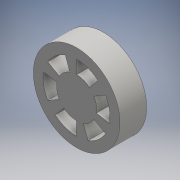
# Autodesk Inventor part: Large Flywheel
Saved by Autodesk Inventor 2016 (Build 200138000, 138)
## iProperties
Created: 2015-12-24
Part Number: Large Flywheel
Material: Generic
Document SubType Name: Modeling
Designer: jonathan
Density: 1 g/cm^3
Appearance: Default
Author: jonathan
Autodesk Inventor part; units mm, degrees
ref_plane "YZ Plane" through (0, 0, 0) normal (1, 0, 0) x (0, 1, 0)
ref_plane "XZ Plane" through (0, 0, 0) normal (0, 1, 0) x (-1, 0, 0)
ref_plane "XY Plane" through (0, 0, 0) normal (0, 0, 1) x (1, 0, 0)
sketch "Sketch1" plane through (0, 0, 0) normal (0, 1, 0) x (-1, 0, 0)
  circle A0 centre (0, 0) radius 65
  dimension "d0" = 130
  constraints: 1 centre point, 1 coincident
  measures "d0" diameter of A0
extrude "Extrusion1" add sketch "Sketch1" along normal blind 40
sketch "Sketch2" plane through (0, 0, 0) normal (0, -1, 0) x (1, 0, 0)
  line L0 (0, 0) -> (0, 50)
  arc A0 (32.1394, 38.3022) -> (0, 50) centre (0, 0) ccw
  arc A1 (19.2836, 22.9813) -> (0, 30) centre (0, 0) ccw
  line L1 (0, 0) -> (19.2836, 22.9813)
  line L2 (32.1394, 38.3022) -> (19.2836, 22.9813)
  dimension "d4" = 40
  dimension "d5" = 30
  dimension "d6" = 50
  constraints: 6 end point, 4 point on circle, 2 centre point, 2 coincident, 1 collinear, 1 point on line, 1 vertical
  measures "d4" angle of L0 L1
  measures "d5" radius of A1
  measures "d6" radius of A0
extrude "Extrusion2" cut sketch "Sketch2" against normal through all contours L0 A0 L2 A1
pattern_circular "Circular Pattern1" count 6 over 360 about axis through (0, 0, 0) along (0, 1, 0) of "Extrusion2"
body "Solid1"
